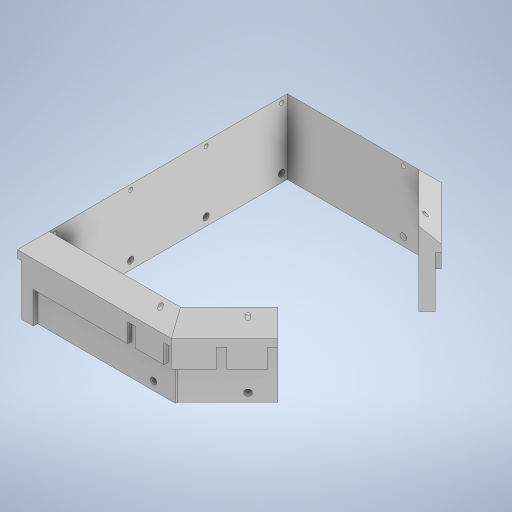
# Autodesk Inventor part: Palm_FingerAttachment
Saved by Autodesk Inventor 2023 (Build 270158000, 158)
## iProperties
Created: 2023-04-19
Part Number: Palm_FingerAttachment
Material: Generic
Document SubType Name: Modeling
Designer: 1senadi
Density: 1 g/cm^3
Appearance: Default
Author: 1senadi
Autodesk Inventor part; units mm, degrees
ref_plane "YZ Plane" through (0, 0, 0) normal (1, 0, 0) x (0, 1, 0)
ref_plane "XZ Plane" through (0, 0, 0) normal (0, 1, 0) x (-1, 0, 0)
ref_plane "XY Plane" through (0, 0, 0) normal (0, 0, 1) x (1, 0, 0)
sketch "Sketch1" plane through (0, 0, 0) normal (0, 1, 0) x (-1, 0, 0)
  line L0 (0, 0) -> (102, 0)
  line L1 (102, 0) -> (102, 127.4)
  line L2 (102, 127.4) -> (0, 127.4)
  line L3 (0, 127.4) -> (0, 0)
  line L4 (94.5, 119.9) -> (94.5, 7.5)
  line L5 (94.5, 7.5) -> (7.5, 7.5)
  line L6 (7.5, 7.5) -> (7.5, 119.9)
  line L7 (7.5, 119.9) -> (94.5, 119.9)
  dimension "d0" = 102
  dimension "d1" = 127.4
  dimension "d2" = 7.5
  constraints: 16 end point, 4 parallel, 2 perpendicular, 1 horizontal, 3 other
  measures "d0" distance of L2.end L1.end
  measures "d1" distance of L1.end L0.end
  measures "d2" distance between parallel lines of L1 L4
extrude "Extrusion1" add sketch "Sketch1" along normal blind 20
sketch "Sketch2" plane through (-102, 0, 0) normal (-1, 0, 0) x (0, 0, 1)
  line L0 (0, 0) -> (0, 9)
  line L1 (0, 0) -> (0, 20) projected
  line L2 (0, 9) -> (3.5, 9)
  line L3 (3.5, 9) -> (3.5, 0)
  line L4 (127.4, 0) -> (0, 0) projected
  line L5 (0, 0) -> (3.5, 0)
  line L6 (3.5, 0) -> (17.1, 0)
  line L7 (17.1, 0) -> (17.1, 9)
  line L8 (17.1, 9) -> (20.6, 9)
  line L9 (20.6, 9) -> (20.6, 0)
  line L10 (17.1, 0) -> (20.6, 0)
  line L11 (56.2, 9) -> (56.2, 0)
  line L12 (52.7, 9) -> (56.2, 9)
  line L13 (52.7, 0) -> (52.7, 9)
  line L14 (52.7, 0) -> (56.2, 0)
  line L15 (39.1, 0) -> (52.7, 0)
  line L16 (39.1, 9) -> (39.1, 0)
  line L17 (35.6, 9) -> (39.1, 9)
  line L18 (35.6, 0) -> (35.6, 9)
  line L19 (35.6, 0) -> (39.1, 0)
  line L20 (91.8, 9) -> (91.8, 0)
  line L21 (88.3, 9) -> (91.8, 9)
  line L22 (88.3, 0) -> (88.3, 9)
  line L23 (88.3, 0) -> (91.8, 0)
  line L24 (74.7, 0) -> (88.3, 0)
  line L25 (74.7, 9) -> (74.7, 0)
  line L26 (71.2, 9) -> (74.7, 9)
  line L27 (71.2, 0) -> (71.2, 9)
  line L28 (71.2, 0) -> (74.7, 0)
  line L29 (106.8, 0) -> (106.8, 9)
  line L30 (106.8, 9) -> (110.3, 9)
  line L31 (123.9, 0) -> (123.9, 9)
  line L32 (127.4, 9) -> (127.4, 0)
  line L33 (123.9, 9) -> (127.4, 9)
  line L34 (110.3, 9) -> (110.3, 0)
  line L35 (106.8, 0) -> (110.3, 0)
  line L36 (110.3, 0) -> (123.9, 0)
  line L37 (123.9, 0) -> (127.4, 0)
  point P0 (88.3, 0)
  point P1 (74.7, 0)
  point P2 (52.7, 0)
  point P3 (39.1, 0)
  point P4 (110.3, 0)
  dimension "d5" = 9
  dimension "d6" = 3.5
  dimension "d7" = 13.6
  dimension "d8" = 9
  dimension "d9" = 3.5
  dimension "d12" = 35.6
  dimension "d222" = 35.6
  constraints: 72 end point, 6 perpendicular, 4 point on line, 2 horizontal, 1 collinear, 51 other
  measures "d5" distance of L0.start L0.end
  measures "d6" distance of L0.end L2.end
  measures "d7" distance of L3.end L6.end
  measures "d8" distance of L6.end L7.end
  measures "d9" distance of L7.end L8.end
  measures "d12" distance of L8.end L11.start
  measures "d222" distance of L27.start L29.start
extrude "Extrusion2" cut sketch "Sketch2" against normal blind 2
sketch "Sketch4" plane through (-102, 20, 127.4) normal (0, 0, 1) x (1, 0, 0)
  line L0 (2, -20) -> (0, -20) projected
  line L1 (2, -20) -> (52, -20)
  line L2 (7.5, -20) -> (94.5, -20) projected
  line L3 (52, -20) -> (52, -11)
  line L4 (52, -11) -> (55.5, -11)
  line L5 (55.5, -11) -> (55.5, -20)
  line L6 (52, -20) -> (55.5, -20)
  line L7 (55.5, -20) -> (69.1, -20)
  line L8 (69.1, -20) -> (69.1, -11)
  line L9 (69.1, -11) -> (72.6, -11)
  line L10 (72.6, -11) -> (72.6, -20)
  line L11 (72.6, -20) -> (69.1, -20)
  point P0 (102, -20)
  dimension "d19" = 50
  dimension "d20" = 9
  dimension "d21" = 3.5
  dimension "d22" = 13.6
  dimension "d23" = 9
  dimension "d24" = 3.5
  constraints: 20 end point, 6 point on line, 3 perpendicular, 2 collinear, 1 vertical
  measures "d19" distance of L0.start L1.end
  measures "d20" distance of L1.end L3.end
  measures "d21" distance of L3.end L4.end
  measures "d22" distance of L5.end L7.end
  measures "d23" distance of L7.end L8.end
  measures "d24" distance of L8.end L9.end
extrude "Extrusion3" cut sketch "Sketch4" against normal blind 2
sketch "Sketch5" plane through (0, 0, 0) normal (0, -1, 0) x (1, 0, 0)
  line L0 (0, 0) -> (-100, 0) projected
  line L1 (0, 127.4) -> (0, 0) projected
  line L2 (-29.4, 127.4) -> (0, 127.4) projected
  line L3 (-29.4, 127.4) -> (-29.4, 125.4) projected
  line L4 (-29.4, 125.4) -> (-32.9, 125.4) projected
  line L5 (-32.9, 125.4) -> (-32.9, 127.4) projected
  line L6 (-46.5, 127.4) -> (-32.9, 127.4) projected
  line L7 (-46.5, 127.4) -> (-46.5, 125.4) projected
  line L8 (-46.5, 125.4) -> (-50, 125.4) projected
  line L9 (-50, 125.4) -> (-50, 127.4) projected
  line L10 (-100, 127.4) -> (-50, 127.4) projected
  line L11 (-100, 127.4) -> (-100, 123.9) projected
  line L12 (-100, 88.3) -> (-102, 88.3) projected
  line L13 (-102, 74.7) -> (-102, 88.3) projected
  line L14 (-102, 74.7) -> (-100, 74.7) projected
  line L15 (-100, 74.7) -> (-100, 71.2) projected
  line L16 (-100, 71.2) -> (-102, 71.2) projected
  line L17 (-102, 56.2) -> (-102, 71.2) projected
  line L18 (-102, 56.2) -> (-100, 56.2) projected
  line L19 (-100, 56.2) -> (-100, 52.7) projected
  line L20 (-100, 52.7) -> (-102, 52.7) projected
  line L21 (-102, 39.1) -> (-102, 52.7) projected
  line L22 (-102, 39.1) -> (-100, 39.1) projected
  line L23 (-100, 39.1) -> (-100, 35.6) projected
  line L24 (-100, 35.6) -> (-102, 35.6) projected
  line L25 (-102, 20.6) -> (-102, 35.6) projected
  line L26 (-102, 20.6) -> (-100, 20.6) projected
  line L27 (-100, 20.6) -> (-100, 17.1) projected
  line L28 (-100, 17.1) -> (-102, 17.1) projected
  line L29 (-102, 3.5) -> (-102, 17.1) projected
  line L30 (-102, 3.5) -> (-100, 3.5) projected
  line L31 (-100, 3.5) -> (-100, 0) projected
  line L32 (-94.5, 119.9) -> (-94.5, 7.5) projected
  line L33 (-7.5, 119.9) -> (-94.5, 119.9) projected
  line L34 (-7.5, 7.5) -> (-7.5, 119.9) projected
  line L35 (-94.5, 7.5) -> (-7.5, 7.5) projected
  line L36 (-59.4, 0) -> (-59.4, 2) projected
  line L37 (-29.4, 127.4) -> (-29.4, 125.4) projected
  line L38 (-102, 127.4) -> (0, 127.4) projected
  line L39 (-29.4, 127.4) -> (0, 127.4)
  line L40 (0, 127.4) -> (0, 0)
  line L41 (-29.4, 0) -> (0, 0)
  line L42 (-29.4, 127.4) -> (-29.4, 0)
  line L43 (0, 0) -> (-102, 0) projected
  line L44 (-29.4, 0) -> (0, 0)
  line L45 (-102, 110.3) -> (-102, 123.9) projected
  line L46 (-102, 91.8) -> (-100, 91.8) projected
  line L47 (-100, 123.9) -> (-102, 123.9) projected
  line L48 (-102, 110.3) -> (-100, 110.3) projected
  line L49 (-100, 110.3) -> (-100, 106.8) projected
  line L50 (-100, 106.8) -> (-102, 106.8) projected
  line L51 (-102, 91.8) -> (-102, 106.8) projected
  line L52 (-100, 91.8) -> (-100, 88.3) projected
  point P0 (-80, 0)
  point P1 (-76.5, 0)
  point P2 (-62.9, 0)
  point P3 (-29.4, 0)
  constraints: 10 end point, 2 collinear, 2 perpendicular, 3 other
extrude "Extrusion4" cut sketch "Sketch5" against normal up to surface (20 mm away) contours L0 L42 L35 L34 L33 L3 L2 L1 | L42 L33 L34 L35
sketch "Sketch6" plane through (-102, 9, 127.4) normal (0, 0, 1) x (1, 0, 0)
  line L0 (0, 11) -> (72.6, 11) projected
  line L1 (0, 11) -> (0, 3.5)
  line L2 (0, 0) -> (0, 11) projected
  line L3 (0, 3.5) -> (7.5, 11)
  line L4 (7.5, 11) -> (0, 11)
  point P0 (102, -9)
  point P1 (42.6, 11)
  point P2 (7.5, 11)
  point P3 (53.613, 11)
  point P4 (2, 11)
  point P5 (0, -9)
  dimension "d29" = 7.5
  dimension "d30" = 45
  constraints: 6 end point, 1 perpendicular, 1 point on line
  measures "d29" distance of L0.start L1.end
  measures "d30" angle of L3 L1
extrude "Extrusion5" cut sketch "Sketch6" against normal up to surface (127.4 mm away)
sketch "Sketch8" plane through (-102, 0, 20.6) normal (-1, 0, 0) x (0, 0, 1)
  line L0 (54.1, 0) -> (67.7, 0) projected
  line L1 (60.9, 0) -> (60.9, 2.75)
  line L2 (60.9, 0) -> (63.65, 0) construction
  circle A0 centre (60.9, 2.75) radius 1.5
  line L3 (60.9, 2.75) -> (60.9, 20)
  line L4 (-20.6, 20) -> (106.8, 20) projected
  line L5 (60.9, 20) -> (60.9, 17.75)
  circle A1 centre (60.9, 17.75) radius 1
  circle A2 centre (25.3, 2.75) radius 1.5
  circle A3 centre (25.3, 17.75) radius 1
  circle A4 centre (-10.3, 2.75) radius 1.5
  circle A5 centre (-10.3, 17.75) radius 1
  circle A6 centre (96.5, 17.75) radius 1
  point P0 (-20.6, 0)
  point P1 (-13.1, 20)
  point P2 (63.7, 20)
  dimension "d38" = 2.75
  dimension "d39" = 90
  dimension "d40" = 3
  dimension "d41" = 2.25
  dimension "d42" = 2
  dimension "d45" = 35.6
  dimension "d229" = 35.6
  constraints: 8 end point, 7 centre point, 3 horizontal, 2 coincident, 2 point on line, 2 vertical, 1 midpoint, 1 perpendicular, 10 other
  measures "d38" distance of L1.start L1.end
  measures "d39" angle of L2 L1
  measures "d40" diameter of A0
  measures "d41" distance of L3.end L5.end
  measures "d42" diameter of A1
  measures "d45" distance of L3.start A2.centre
  measures "d229" distance of A1.centre A6.centre
extrude "Extrusion7" cut sketch "Sketch8" against normal up to surface (7.5 mm away) contours A1 L3 | L3 A1 | A3 | A5 | A6
sketch "Sketch35" plane through (-100, 9, 0) normal (0, 0, -1) x (-1, 0, 0)
  line L0 (0, -9) -> (-50, -9) projected
  line L1 (-5.5, -9) -> (0, -9)
  line L2 (0, -9) -> (0, -24)
  line L3 (0, 0) -> (0, -9) projected
  line L4 (-5.5, -9) -> (-5.5, 11) projected
  line L5 (-5.5, -9) -> (-5.5, -24)
  line L6 (-5.5, -9) -> (9.5, -9) construction
  line L7 (-5.5, -24) -> (0, -24)
  point P0 (-100, -9)
  point P1 (2, -9)
  dimension "d215" = 15
  dimension "d216" = 15
  dimension "d217" = 90
  constraints: 10 end point, 3 collinear, 1 horizontal, 1 perpendicular
  measures "d215" distance of L0.start L2.end
  measures "d216" distance of L1.start L5.end
  measures "d217" angle of L5 L6
extrude "Extrusion28" add sketch "Sketch35" against normal up to surface (127.4 mm away)
sketch "Sketch36" plane through (-100, 0, 0) normal (-1, 0, 0) x (0, 0, 1)
  line L0 (3.5, 0) -> (17.1, 0) projected
  line L1 (10.3, 0) -> (10.3, -15)
  line L2 (0, -15) -> (127.4, -15) projected
  line L3 (10.3, -15) -> (10.3, -11)
  circle A0 centre (10.3, -11) radius 1.5
  circle A1 centre (45.9, -11) radius 1.5
  circle A2 centre (81.5, -11) radius 1.5
  circle A3 centre (117.1, -11) radius 1.5
  point P0 (0, 0)
  dimension "d234" = 4
  dimension "d235" = 3
  dimension "d238" = 35.6
  constraints: 4 centre point, 4 end point, 2 point on line, 1 coincident, 1 horizontal, 1 midpoint, 1 vertical, 6 other
  measures "d234" distance of L1.end L3.end
  measures "d235" diameter of A0
  measures "d238" distance of A0.centre A1.centre
extrude "Extrusion29" cut sketch "Sketch36" against normal up to surface (5.5 mm away)
ref_plane "Work Plane5" through (-102, 0, 63.7) normal (0, 0, 1) x (1, 0, 0)
mirror "Mirror7" about plane through (-102, 0, 63.7) normal (0, 0, 1) of "Extrusion3"
sketch "Sketch37" plane through (-94.5, 0, 127.4) normal (1, 0, 0) x (0, 0, -1)
  line L0 (7.5, 0) -> (2, 0) projected
  line L1 (2, 0) -> (2, -15)
  line L2 (127.4, -15) -> (0, -15) projected
  line L3 (7.5, 0) -> (7.5, -15)
  line L4 (7.5, -15) -> (2, -15)
  line L5 (7.5, 0) -> (2, 0)
  line L6 (127.4, 0) -> (119.9, 0) projected
  line L7 (125.4, 0) -> (125.4, -15)
  line L8 (119.9, 0) -> (119.9, -15)
  line L9 (125.4, -15) -> (119.9, -15)
  constraints: 14 end point, 4 point on line, 3 collinear, 3 perpendicular, 1 vertical
extrude "Extrusion30" add sketch "Sketch37" along normal up to surface (65.1 mm away)
sketch "Sketch39" plane through (0, 20, 0) normal (0, 1, 0) x (1, 0, 0)
  line L0 (-29.4, -7.5) -> (-29.4, 0) projected
  line L1 (-29.4, 0) -> (-4.227, -25.173)
  line L2 (-29.4, 0) -> (6.2, 0) construction
  line L3 (-4.227, -25.173) -> (-9.5303, -30.4763)
  line L4 (-9.5303, -30.4763) -> (-32.5066, -7.5)
  line L5 (-94.5, -7.5) -> (-29.4, -7.5) projected
  point P0 (0, 0)
  dimension "d247" = 35.6
  dimension "d248" = 45
  dimension "d249" = 7.5
  dimension "d250" = 90
  constraints: 8 end point, 2 perpendicular, 1 equal length, 1 horizontal, 1 point on line
  measures "d247" distance of L0.end L1.end
  measures "d248" angle of L1 L2
  measures "d249" distance of L1.end L3.end
  measures "d250" angle of L1 L3
extrude "Extrusion31" add sketch "Sketch39" against normal up to surface (20 mm away)
sketch "Sketch41" plane through (-4.227, 0, 25.173) normal (0.7071068, 0, -0.7071068) x (-0.7071068, 0, -0.7071068)
  line L0 (35.6, 0) -> (0, 0) projected
  line L1 (35.6, 0) -> (0, 0) projected
  line L2 (35.6, 9) -> (35.6, 0) projected
  line L3 (35.6, 20) -> (35.6, 9) projected
  line L4 (0, 20) -> (35.6, 20) projected
  line L5 (0, 20) -> (0, 0) projected
  line L6 (0, 0) -> (0, 9)
  line L7 (0, 20) -> (0, 0) projected
  line L8 (0, 9) -> (3.5, 9)
  line L9 (3.5, 9) -> (3.5, 0)
  line L10 (7.5279, 0) -> (-2.0888, 0) projected
  line L11 (0, 0) -> (3.5, 0)
  line L12 (3.5, 0) -> (17.1, 0)
  line L13 (17.1, 0) -> (17.1, 9)
  line L14 (17.1, 9) -> (20.6, 9)
  line L15 (20.6, 9) -> (20.6, 0)
  line L16 (22.0235, 0) -> (11.4169, 0) projected
  line L17 (17.1, 0) -> (20.6, 0)
  point P0 (14.8111, 0)
  point P1 (3.5, 0)
  point P2 (0, 0)
  dimension "d253" = 9
  dimension "d254" = 3.5
  dimension "d255" = 90
  dimension "d256" = 13.6
  dimension "d257" = 9
  dimension "d258" = 3.5
  constraints: 18 end point, 6 point on line, 3 perpendicular, 2 collinear
  measures "d253" distance of L1.end L6.end
  measures "d254" distance of L6.end L8.end
  measures "d255" angle of L6 L8
  measures "d256" distance of L9.end L12.end
  measures "d257" distance of L12.end L13.end
  measures "d258" distance of L13.end L14.end
extrude "Extrusion32" cut sketch "Sketch41" against normal blind 2 contours L0 L13 L14 L15 | L8 L9 L0 L5
sketch "Sketch42" plane through (-100, -15, 0) normal (0, -1, 0) x (1, 0, 0)
  line L0 (70.6, 7.5) -> (67.4934, 7.5) projected
  line L1 (90.4697, 30.4763) -> (67.4934, 7.5) projected
  line L2 (67.4934, 7.5) -> (90.4697, 30.4763)
  line L3 (91.8839, 24.1123) -> (94.3588, 26.5872) projected
  line L4 (90.4697, 30.4763) -> (94.3588, 26.5872)
  line L5 (90.4697, 30.4763) -> (95.773, 25.173) projected
  line L6 (70.6, 2) -> (70.6, 7.5) projected
  line L7 (79.7924, 12.0208) -> (82.2673, 14.4957) projected
  line L8 (94.3588, 26.5872) -> (95.773, 25.173) projected
  line L9 (94.3588, 26.5872) -> (70.6, 2.8284)
  point P0 (100, 0)
  constraints: 6 end point, 2 collinear, 1 point on line
extrude "Extrusion33" add sketch "Sketch42" against normal up to surface (15 mm away)
sketch "Sketch43" plane through (-29.4, -15, 2) normal (0, 0, -1) x (-1, 0, 0)
  line L0 (17.1, 15) -> (3.5, 15) projected
  line L1 (10.3, 15) -> (10.3, 0)
  line L2 (65.1, 0) -> (3.1066, 0) projected
  line L3 (10.3, 0) -> (10.3, 4)
  circle A0 centre (10.3, 4) radius 1.5
  point P0 (-29.4, 15)
  dimension "d263" = 4
  dimension "d264" = 3
  constraints: 4 end point, 2 point on line, 1 centre point, 1 coincident, 1 midpoint, 1 vertical
  measures "d263" distance of L1.end L3.end
  measures "d264" diameter of A0
extrude "Extrusion34" cut sketch "Sketch43" against normal up to surface (5.5 mm away)
sketch "Sketch44" plane through (-5.6412, 0, 26.5872) normal (0.7071068, 0, -0.7071068) x (-0.7071068, 0, -0.7071068)
  line L0 (10.0027, 0) -> (10.0027, 9) projected
  line L1 (10.0027, 0) -> (10.0027, -15)
  line L2 (76.3294, -15) -> (-3.1495, -15) projected
  line L3 (10.0027, -15) -> (10.0027, -11)
  circle A0 centre (10.0027, -11) radius 1.5
  point P0 (14.8111, 0)
  dimension "d267" = 4
  dimension "d268" = 3
  constraints: 4 end point, 2 point on line, 1 centre point, 1 coincident, 1 vertical
  measures "d267" distance of L1.end L3.end
  measures "d268" diameter of A0
extrude "Extrusion35" cut sketch "Sketch44" against normal up to surface (5.5 mm away)
sketch "Sketch45" plane through (-9.5303, -15, 30.4763) normal (0.7071068, 0, 0.7071068) x (0.7071068, 0, -0.7071068)
  line L0 (7.5, 35) -> (7.5, 24) projected
  line L1 (7.5, 35) -> (7.5, 27.5)
  line L2 (0, 0) -> (0, 35) projected
  line L3 (7.5, 27.5) -> (0, 35)
  line L4 (0, 35) -> (7.5, 35)
  point P0 (28.2889, 15)
  dimension "d271" = 7.5
  dimension "d272" = 45
  constraints: 6 end point, 1 perpendicular, 1 point on line
  measures "d271" distance of L0.start L1.end
  measures "d272" angle of L1 L3
extrude "Extrusion36" cut sketch "Sketch45" against normal up to surface (35.6 mm away)
ref_plane "Work Plane6" through (-29.4, 20, 119.9) normal (1, 0, 0) x (0, 0, -1)
sketch "Sketch46" plane through (-29.4, 20, 119.9) normal (1, 0, 0) x (0, 0, -1)
  line L0 (119.9, -7.5) -> (119.9, 0) projected
  line L1 (119.9, 0) -> (119.9, -7.5)
  line L2 (119.9, 0) -> (112.4, 0) projected
  line L3 (119.9, -7.5) -> (112.4, 0)
  line L4 (112.4, 0) -> (119.9, 0)
  point P0 (119.9, -20)
  dimension "d276" = 45
  constraints: 6 end point, 1 collinear, 1 vertical
  measures "d276" angle of L1 L3
extrude "Extrusion37" cut sketch "Sketch46" against normal up to surface (72.6 mm away)
sketch "Sketch47" plane through (-94.5, -15, 0) normal (0, 0, -1) x (-1, 0, 0)
  line L0 (-61.6, 15) -> (-48, 15) projected
  line L1 (-54.8, 15) -> (-54.8, 35)
  line L2 (0, 35) -> (-61.9934, 35) projected
  line L3 (-54.8, 35) -> (-54.8, 32.75)
  circle A0 centre (-54.8, 32.75) radius 1
  point P0 (-94.5, 15)
  dimension "d279" = 2.25
  dimension "d280" = 2
  constraints: 4 end point, 2 point on line, 1 centre point, 1 coincident, 1 midpoint, 1 vertical
  measures "d279" distance of L1.end L3.end
  measures "d280" diameter of A0
extrude "Extrusion38" cut sketch "Sketch47" against normal up to surface (7.5 mm away)
sketch "Sketch48" plane through (-29.4, 0, 0) normal (0.7071068, 0, -0.7071068) x (-0.7071068, 0, -0.7071068)
  line L0 (-3.1066, 20) -> (-35.6, 20) projected
  line L1 (-25.5973, 0) -> (-24.1831, 0) projected
  line L2 (-25.5973, 0) -> (-25.5973, 20)
  line L3 (-25.5973, 20) -> (-25.5973, 17.75)
  line L4 (-25.5973, 20) -> (-23.3473, 20) construction
  circle A0 centre (-25.5973, 17.75) radius 1
  point P0 (-20.7889, 0)
  dimension "d283" = 2.25
  dimension "d284" = 90
  dimension "d285" = 2
  constraints: 6 end point, 2 perpendicular, 1 centre point, 1 coincident, 1 collinear, 1 horizontal, 1 point on line
  measures "d283" distance of L2.end L3.end
  measures "d284" angle of L3 L4
  measures "d285" diameter of A0
extrude "Extrusion39" cut sketch "Sketch48" against normal up to surface (7.5 mm away)
mirror "Mirror10" about plane through (-102, 0, 63.7) normal (0, 0, 1) of "Extrusion36", "Extrusion37", "Extrusion38", "Extrusion39", "Extrusion32", "Extrusion35", "Extrusion3", "Mirror7", "Extrusion34", "Extrusion33", "Extrusion31"
body "Solid1"
